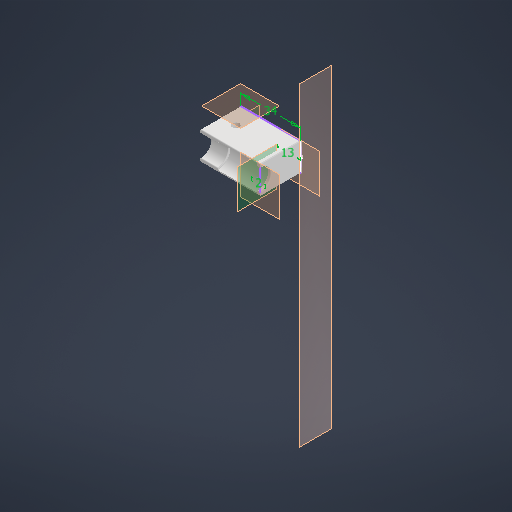
# Autodesk Inventor part: thermoMETER_mount
Saved by Autodesk Inventor 2027.1 (Build 311270010, 270A)
## iProperties
Created: 2026-09-09
Part Number: thermoMETER_mount
Material: Generic
Document SubType Name: Modeling
Designer: Jacob Parker
Density: 1 g/cm^3
Appearance: Default
Author: Jacob Parker
Autodesk Inventor part; units mm, degrees
ref_plane "YZ Plane" through (0, 0, 0) normal (1, 0, 0) x (0, 1, 0)
ref_plane "XZ Plane" through (0, 0, 0) normal (0, 1, 0) x (-1, 0, 0)
ref_plane "Work Plane1" through (55, -127.943, -12.5) normal (1, 0, 0) x (0, 0, -1)
ref_plane "Work Plane2" through (2, 0, 0) normal (1, 0, 0) x (0, 1, 0)
ref_plane "Work Plane8" through (55, 3.2, 4) normal (0, 0, 1) x (1, 0, 0)
sketch "SKbody" plane through (55, 3.2, 4) normal (0, 0, 1) x (1, 0, 0)
  line L0 (0, 10.8) -> (-34, 10.8)
  line L1 (-34, -5.2) -> (0, -5.2)
  line L2 (-34, 10.8) -> (-34, -5.2)
  line L3 (0, -5.2) -> (0, 10.8)
  line L4 (0, -2.2986) -> (0, 7.8986)
  point P0 (-13, 2.8)
  point P1 (0, 2.8)
  dimension "d19" = 34
  dimension "d20" = 13
  constraints: 10 end point, 1 collinear, 1 midpoint, 2 other
  measures "d19" distance of L0.start L0.end
  measures "d20" distance of point (-13, 2.8) point (0, 2.8)
extrude "EXbody" add sketch "SKbody" along normal blind 22.8
ref_plane "Work Plane6" through (21, -2, 4) normal (-1, 0, 0) x (0, 0, 1)
sketch "SKhole1" plane through (21, -2, 4) normal (-1, 0, 0) x (0, 0, 1)
  line L0 (22.8, 16) -> (22.8, 0)
  circle A0 centre (22.8, 8) radius 6
  point P0 (22.8, 2)
  point P1 (22.8, 14)
  dimension "d11" = 12
  constraints: 2 end point, 1 centre point, 1 midpoint
  measures "d11" diameter of A0
extrude "EXhole1" cut sketch "SKhole1" against normal through all contours L0 A0 picked at (20.93, 8.7092)
ref_plane "Work Plane5" through (55, 3.2, 26.8) normal (0, 0, 1) x (1, 0, 0)
sketch "SKplaneref" plane through (55, 3.2, 26.8) normal (0, 0, 1) x (1, 0, 0)
  line L0 (0, 8.8) -> (0, -3.2)
  line L1 (0, 2.8) -> (-2, 2.8)
  dimension "d15" = 2
  constraints: 4 end point, 1 horizontal, 1 midpoint
  measures "d15" distance of L1.start L1.end
ref_plane "Work Plane3" through (53, 6, 26.8) normal (-1, 0, 0) x (0, -1, 0)
sketch "SKhole2" plane through (53, 6, 26.8) normal (-1, 0, 0) x (0, -1, 0)
  arc A0 (-6, 0) -> (6, 0) centre (0, 0) ccw projected
  circle A1 centre (0, 0) radius 7
  point P0 (6, -26.8)
  dimension "d16" = 14
  constraints: 1 centre point, 1 coincident
  measures "d16" diameter of A1
extrude "EXhole2" cut sketch "SKhole2" along normal blind 22
ref_plane "Work Plane7" through (21, 14, 4) normal (0, 1, 0) x (1, 0, 0)
sketch "SKziptiehole" plane through (21, 14, 4) normal (0, 1, 0) x (1, 0, 0)
  line L0 (34, -22.8) -> (0, -22.8)
  line L1 (0, 0) -> (0, -22.8)
  point P0 (8, -10.8)
  dimension "d42" = 12
  dimension "d43" = 8
  constraints: 4 end point
  measures "d42" distance from line of L0 point (8, -10.8)
  measures "d43" distance from line of L1 point (8, -10.8)
hole "Hziptiehole" at (29, 14, 14.8) direction (0, -1, 0) diameter 4 end through all
fillet "Fillet1" radius 0.5 12 edges at (21, 14, 15.4) (38, 14, 26.8) (38, -2, 26.8) (21, -2, 15.4) (55, 14, 15.4) (55, -2, 15.4) (55, 6, 20.8) (21, 6, 20.8) (26, 0, 26.8) (26, 12, 26.8) (53, 6, 20.8) (31, 6, 20.8)
body "Solid1"
